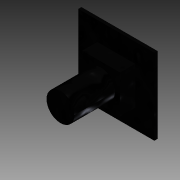
# Autodesk Inventor part: Camera
Saved by Autodesk Inventor 2013 (Build 170138000, 138)
## iProperties
Created: 2014-08-02
Part Number: Camera
Material: ABS Plastic
Document SubType Name: Modeling
Designer: Kyle
Density: 1 g/cm^3
Author: Kyle
Autodesk Inventor part; units mm, degrees
ref_plane "YZ Plane" through (0, 0, 0) normal (1, 0, 0) x (0, 1, 0)
ref_plane "XZ Plane" through (0, 0, 0) normal (0, 1, 0) x (-1, 0, 0)
ref_plane "XY Plane" through (0, 0, 0) normal (0, 0, 1) x (1, 0, 0)
sketch "Sketch1" plane through (0, 0, 0) normal (0, 0, 1) x (1, 0, 0)
  line L0 (0, 0) -> (38.1, 0)
  line L1 (38.1, 0) -> (38.1, -38.1)
  line L2 (38.1, -38.1) -> (0, -38.1)
  line L3 (0, -38.1) -> (0, 0)
  dimension "d0" = 38.1
  dimension "d1" = 38.1
  constraints: 8 end point, 2 parallel, 1 horizontal, 1 perpendicular
  measures "d0" distance of L0.start L0.end
  measures "d1" distance of L2.end L0.start
extrude "Extrusion1" add sketch "Sketch1" along normal blind 1.6002
sketch "Sketch2" plane through (0, 0, 1.6002) normal (0, 0, 1) x (1, 0, 0)
  line L0 (38.1, 0) -> (0, 0) projected
  line L1 (0, 0) -> (0, -38.1) projected
  line L2 (0, -38.1) -> (38.1, -38.1) projected
  line L3 (38.1, -38.1) -> (38.1, 0) projected
  line L4 (9.525, -9.525) -> (28.575, -9.525)
  line L5 (28.575, -9.525) -> (28.575, -28.575)
  line L6 (28.575, -28.575) -> (9.525, -28.575)
  line L7 (9.525, -28.575) -> (9.525, -9.525)
  dimension "d4" = 9.525
  dimension "d5" = 9.525
  dimension "d6" = 9.525
  dimension "d7" = 9.525
  constraints: 8 end point, 2 parallel, 1 horizontal, 1 perpendicular
  measures "d4" distance between parallel lines of L0 L4
  measures "d5" distance between parallel lines of L3 L5
  measures "d6" distance between parallel lines of L2 L6
  measures "d7" distance between parallel lines of L1 L7
extrude "Extrusion2" add sketch "Sketch2" along normal blind 7.62 contours L4 L5 L6 L7
sketch "Sketch3" plane through (0, 0, 9.2202) normal (0, 0, 1) x (1, 0, 0)
  circle A0 centre (19.05, -19.05) radius 6.985
  point P0 (0, 0)
  dimension "d10" = 13.97
  constraints: 1 centre point, 1 coincident, 1 other
  measures "d10" diameter of A0
extrude "Extrusion3" add sketch "Sketch3" along normal blind 20.32
body "Solid1"
